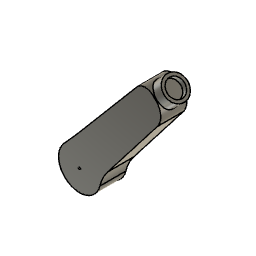
robot arm v3 (Autodesk Fusion 360 archive; units mm, degrees)
design "arm 2"
Autodesk Fusion 360 part; units mm, degrees
sketch "Sketch1" plane through (0, 0, 0) normal (0, 1, 0) x (1, 0, 0)
  circle A0 centre (0, 0) radius 19.355
  dimension "d1" = 38.71
  constraint coincident A0.centre origin
  measures "d1" diameter of A0
extrude "Extrude1" add sketch "Sketch1" along normal blind 24
sketch "Sketch2" plane through (0, 0, 0) normal (0, -1, 0) x (1, 0, 0)
  circle A0 centre (0, 0) radius 19.355
  line L0 (-11.3182, 15.7008) -> (60, 100)
  line L1 (60, 100) -> (80, 80)
  line L2 (80, 80) -> (19.2899, 1.5864)
  constraint coincident A0 L0.start
  constraint coincident A0 L2.end
extrude "Extrude2" add sketch "Sketch2" against normal blind 24 contours A0 L0 L1 L2
sketch "Sketch3" plane through (0, 0, 0) normal (0, -1, 0) x (1, 0, 0)
  arc A0 (-11.3182, 15.7008) -> (19.2899, 1.5864) centre (0, 0) ccw
  line L0 (19.2899, 1.5864) -> (80, 80)
  line L1 (80, 80) -> (60, 100)
  line L2 (60, 100) -> (-11.3182, 15.7008)
  constraint coincident A0.centre origin
hole "Hole1" at (0, 0, 0) direction (0, 1, 0) diameter 2 depth 10 tip angle 180 counterbore diameter 2 counterbore depth 10
sketch "Sketch4" plane through (80, 0, 80) normal (0.707107, 0, 0.707107) x (0, 1, 0)
  line L0 (0, 28.2843) -> (0, 0)
  line L1 (0, 0) -> (24, 0)
  line L2 (24, 0) -> (24, 28.2843)
  line L3 (24, 28.2843) -> (0, 28.2843)
  circle A0 centre (11.8031, 14.1421) radius 10.9673
extrude "Extrude3" add sketch "Sketch4" along normal blind 10 contours A0
sketch "Sketch5" plane through (87.0711, 0, 87.0711) normal (0.707107, 0, 0.707107) x (0, 1, 0)
  circle A0 centre (11.8031, 14.1421) radius 10.9673
  circle A1 centre (11.8031, 14.1421) radius 8.1417
  constraint concentric A0 A1
extrude "Extrude4" cut sketch "Sketch5" against normal blind 5 contours A1
fillet "Fillet1" radius 15 1 edges at (80, 12, 80)
fillet "Fillet2" radius 10 1 edges at (60, 12, 100)
fillet "Fillet3" radius 40 1 edges at (19.2899, 12, 1.5864)
fillet "Fillet4" radius 510 1 edges at (-11.3182, 12, 15.7008)

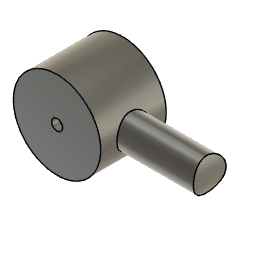
design "joint 5"
Autodesk Fusion 360 part; units mm, degrees
cylinder "CylinderPrimitive1" add diameter 30 height 70 placed x (1, 0, 0) y (0, 1, 0) z (0, 0, 1) at (0, 0, 0) makes body 1
sketch "Sketch2" plane through (0, 0, 0) normal (1, 0, 0) x (0, 1, 0)
sketch "Sketch3" plane through (0, 0, 0) normal (0, 1, 0) x (1, 0, 0)
sketch "Sketch4" plane through (0, 0, 70) normal (0, 0, 1) x (-1, 0, 0)
  circle A0 centre (0, 0) radius 15
  circle A1 centre (0, 0) radius 7.0711
  circle A2 centre (0, 0) radius 9.2041
  constraint concentric A0 A1
  constraint coincident A0.centre A1.centre
extrude "Extrude1" add sketch "Sketch4" along normal blind 5 contours A2 bodies 1
fillet "Fillet1" radius 15 1 edges at (-13.9849, 5.4242, 0) on bodies 1
delete_face "DeleteFace1" 1 faces at (14.9814, -0.7477, 33.3333) on bodies 1
delete_face "DeleteFace2" 1 faces at (14.2211, 3.5457, 18.1918) on bodies 1
sketch "Sketch5" plane through (0, 0, 0) normal (0, 0, 1) x (1, 0, 0)
sketch "Sketch6" plane through (0, 0, 0) normal (0, 1, 0) x (1, 0, 0)
  circle A0 centre (0, 0) radius 20
  dimension "d6" = 40
  constraint coincident A0.centre origin
  measures "d6" diameter of A0
extrude "Extrude2" add sketch "Sketch6" along normal blind 30 separate body makes body 2
sketch "Sketch7" plane through (0, 0, 0) normal (0, -1, 0) x (1, 0, 0)
  circle A0 centre (0, 0) radius 20
sketch "Sketch8" plane through (0, 30, 0) normal (0, 1, 0) x (-1, 0, 0)
  circle A0 centre (0, 0) radius 20
sketch "Sketch9" plane through (0, 0, 0) normal (1, 0, 0) x (0, 1, 0)
  circle A0 centre (14.965, -0.2661) radius 7.5
  dimension "d9" = 15
  measures "d9" diameter of A0
extrude "Extrude3" add sketch "Sketch9" along normal blind 35 from the near side of the face at (19.9006, 20, 1.9914) on bodies 2 bodies 2
sketch "Sketch10" plane through (0, 0, 0) normal (0, 1, 0) x (1, 0, 0)
sketch "Sketch11" plane through (0, 0, 0) normal (0, 1, 0) x (1, 0, 0)
sketch "Sketch12" plane through (0, 0, 0) normal (0, 0, 1) x (1, 0, 0)
sketch "Sketch13" plane through (0, 0, 0) normal (0, -1, 0) x (1, 0, 0)
hole "Hole1" at (0, 0, 0) direction (0, 1, 0) diameter 5 depth 5 tip angle 180 bodies 2
sketch "Sketch14" plane through (0, 30, 0) normal (0, 1, 0) x (-1, 0, 0)
hole "Hole2" at (0, 30, 0) direction (0, -1, 0) diameter 5 depth 5 tip angle 180 bodies 2

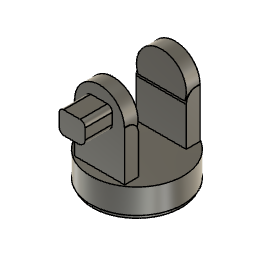
design "first joint"
Autodesk Fusion 360 part; units mm, degrees
sketch "Sketch1" plane through (0, 0, 0) normal (0, 0, 1) x (1, 0, 0)
  circle A0 centre (0, 0) radius 37.5
  dimension "d1" = 75
  constraint coincident A0.centre origin
  measures "d1" diameter of A0
extrude "Extrude1" add sketch "Sketch1" along normal blind 20
sketch "Sketch2" plane through (0, 0, 0) normal (0, 0, -1) x (1, 0, 0)
  circle A0 centre (0, 0) radius 37.5
  circle A1 centre (0, 0) radius 36
  dimension "d4" = 72
  constraint coincident A0.centre A1.centre
  measures "d4" diameter of A1
extrude "Extrude2" add sketch "Sketch2" along normal blind 3 contours A1
sketch "Sketch3" plane through (0, 0, 20) normal (0, 0, 1) x (-1, 0, 0)
  circle A0 centre (0, 0) radius 37.5
  line L0 (20.6675, -31.2906) -> (-20, -31.2906)
  line L1 (-20, -31.2906) -> (-20, -20)
  line L2 (-20, -20) -> (20.6675, -20)
  line L3 (20.6675, -20) -> (20.6675, -31.2906)
  constraint horizontal L0
  constraint vertical L1
  constraint horizontal L2
  constraint vertical L3
  constraint coincident A0 L0.start
extrude "Extrude3" add sketch "Sketch3" along normal blind 40 contours L0 L1 L2 L3
pattern_linear "R-Pattern1" count 2 spacing 50 along (0, -1, 0) of "Extrude3"
sketch "Sketch4" plane through (0, -30, 0) normal (0, -1, 0) x (1, 0, 0)
  line L0 (-20.6675, 20) -> (20, 20)
  line L1 (20, 20) -> (20, 60)
  line L2 (20, 60) -> (-20.6675, 60)
  line L3 (-20.6675, 60) -> (-20.6675, 20)
  circle A0 centre (-0.3338, 60) radius 20.127
  constraint midpoint L2 A0.centre
extrude "Extrude4" add sketch "Sketch4" against normal blind 11.1234 contours L2 A0 picked at (6.0089, 64.8884)
sketch "Sketch5" plane through (0, 31.2906, 0) normal (0, 1, 0) x (-1, 0, 0)
  line L0 (-20, 20) -> (20.6675, 20)
  line L1 (20.6675, 20) -> (20.6675, 60)
  line L2 (20.6675, 60) -> (-20, 60)
  line L3 (-20, 60) -> (-20, 20)
  circle A0 centre (0.3338, 60) radius 20.1945
  constraint midpoint L2 A0.centre
extrude "Extrude5" add sketch "Sketch5" against normal blind 11.134 contours L2 A0 picked at (4.9007, 69.4834)
sketch "Sketch6" plane through (0, -30, 0) normal (0, -1, 0) x (1, 0, 0)
  line L0 (-20.6675, 20) -> (20, 20)
  line L1 (20, 20) -> (20, 60)
  line L2 (20, 60) -> (19.7932, 60)
  arc A0 (19.7932, 60) -> (-20.4607, 60) centre (-0.3338, 60) ccw
  line L3 (-20.4607, 60) -> (-20.6675, 60)
  line L4 (-20.6675, 60) -> (-20.6675, 20)
  line L5 (-11, 70) -> (10, 70)
  line L6 (10, 70) -> (10, 52)
  line L7 (10, 52) -> (-11, 52)
  line L8 (-11, 52) -> (-11, 70)
  constraint horizontal L5
  constraint vertical L6
  constraint horizontal L7
  constraint vertical L8
extrude "Extrude6" add sketch "Sketch6" along normal blind 22 contours L5 L6 L7 L8
fillet "Fillet1" radius 8.5 1 edges at (-0.3338, 20, 60)
fillet "Fillet2" radius 9 1 edges at (-0.3338, -18.7094, 60)
fillet "Fillet3" radius 3.5 1 edges at (-11, -41, 70)
fillet "Fillet4" radius 4 1 edges at (10, -41, 70)
fillet "Fillet5" radius 4 1 edges at (-11, -41, 52)
fillet "Fillet6" radius 5.5 1 edges at (10, -41, 52)
